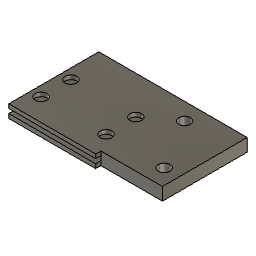
Schleppketten_Adapter_X_top (Autodesk Fusion 360 design; units mm, degrees)
Autodesk Fusion 360 part; units mm, degrees
sketch "Sketch1" plane through (0, 0, 0) normal (0, 0, 1) x (1, 0, 0)
  line L0 (0, 0) -> (41, 0)
  line L1 (41, 0) -> (41, 35)
  line L2 (41, 35) -> (0, 35)
  line L3 (0, 35) -> (0, 0)
  line L4 (0, 17.5) -> (41, 17.5) construction
  circle A0 centre (4.8, 24.5) radius 2.75
  circle A1 centre (4.8, 10.5) radius 2.75
  line L5 (4.8, 24.5) -> (4.8, 10.5) construction
  line L6 (2.05, 10.5) -> (4.8, 10.5) construction
  line L7 (41, 42.475) -> (70, 42.475)
  line L8 (70, 42.475) -> (70, 2.475)
  line L9 (70, 2.475) -> (41, 2.475)
  line L10 (41, 2.475) -> (41, 0)
  line L11 (48.5, 34.45) -> (48.5, 10.5) construction
  circle A2 centre (48.5, 34.45) radius 2.75
  circle A3 centre (48.5, 10.5) radius 2.75 construction
  line L12 (70, 22.475) -> (48.5, 22.475) construction
  line L13 (41, 42.475) -> (41, 35)
  line L14 (0, 35) -> (0, 42.475)
  line L15 (0, 42.475) -> (41, 42.475)
  line L16 (62.8, 34.45) -> (62.8, 10.5) construction
  circle A4 centre (62.8, 34.45) radius 2.75 construction
  circle A5 centre (62.8, 10.5) radius 2.75
  line L17 (48.5, 34.45) -> (62.8, 34.45) construction
  line L18 (48.5, 10.5) -> (62.8, 10.5) construction
  line L19 (35.4, 24.5) -> (35.4, 10.5) construction
  circle A6 centre (35.4, 24.5) radius 2.75
  circle A7 centre (35.4, 10.5) radius 2.75
  point P0 (2.05, 10.5)
  dimension "d1" = 41
  dimension "d2" = 35
  dimension "d3" = 14
  dimension "d7" = 40
  dimension "d8" = 7.5
  dimension "d9" = 5.5
  dimension "d12" = 23.95
  dimension "d13" = 4.8
  dimension "d14" = 5.5
  dimension "d20" = 14.3
  dimension "d21" = 30.6
  dimension "d22" = 29
  constraint horizontal L0
  constraint vertical L1
  constraint horizontal L2
  constraint vertical L3
  constraint coincident L0.start L3.end
  constraint midpoint L3 L4.start
  constraint coincident A0.centre L5.start
  constraint coincident A1.centre L5.end
  constraint perpendicular L4 L5
  constraint symmetric L4 A0.centre A1.centre
  constraint coincident A1 P0
  constraint coincident P0 L6.start
  constraint horizontal L6
  constraint equal A0 A1
  constraint coincident L1 L7.start
  constraint perpendicular L7 L8
  constraint coincident L0 L1.start
  constraint vertical L10
  constraint horizontal L9
  constraint perpendicular L2 L11
  constraint coincident L11.start A2.centre
  constraint coincident L11.end A3.centre
  constraint equal A2 A3
  constraint horizontal L7
  constraint midpoint L8 L12.start
  constraint midpoint L11 L12.end
  constraint horizontal L12
  constraint horizontal L4
  constraint coincident L1 L4.end
  constraint coincident L0.end L10
  constraint perpendicular L2 L14
  constraint horizontal L15
  constraint vertical L16
  constraint equal L11 L16
  constraint coincident L16.start A4.centre
  constraint coincident L16.end A5.centre
  constraint equal A2 A4
  constraint equal A4 A5
  constraint symmetric L12 L16.start L16.end
  constraint coincident A1.centre L18
  constraint perpendicular L9 L19
  constraint symmetric L4 L19.start L19.end
  constraint equal L5 L19
  constraint coincident L19.start A6.centre
  constraint coincident L19.end A7.centre
  constraint equal A6 A7
  constraint equal A0 A6
  measures "d1" distance of L0.start L0.end
  measures "d2" distance of L0.end L1.end
  measures "d3" distance of A0.centre A1.centre
  measures "d7" distance of L7.end L8.end
  measures "d8" distance of L4.end L11
  measures "d9" diameter of A2
  measures "d12" distance of L11.start L11.end
  measures "d13" horizontal distance of L0.start A1.centre
  measures "d14" diameter of A1
  measures "d20" horizontal distance of L11.start L16.start
  measures "d21" distance of A1.centre L19.end
  measures "d22" distance of L8.end L9.end
extrude "Extrude1" add sketch "Sketch1" along normal blind 6
extrude "Extrude2" cut sketch "Sketch1" along normal blind 2.1 from surface at 2 contours L0 L1 L2 L3 L10
equation "d3 = ( ( 9 + 19 ) / 2 ) * 1 mm"
equation "d8 = ( ( 4 + 11 ) / 2 ) * 1 mm"
equation "d12 = ( ( 17.5 + 30.4 ) / 2 ) * 1 mm"
equation "d15 = 2 mm + 2 mm + 2 mm"
equation "d20 = ( 18.3 mm - 4 mm )"
equation "d21 = ( ( 25.6 + 35.6 ) / 2 ) * 1 mm"
